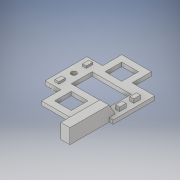
# Autodesk Inventor part: y-axis motor mount modified
Saved by Autodesk Inventor 2018 (Build 220112000, 112)
## iProperties
Created: 2018-02-05
Part Number: y-axis motor mount modified
Material: Generic
Document SubType Name: Modeling
Designer: junai
Density: 1 g/cm^3
Appearance: Default
Author: junai
Autodesk Inventor part; units mm, degrees
ref_plane "YZ Plane" through (0, 0, 0) normal (1, 0, 0) x (0, 1, 0)
ref_plane "XZ Plane" through (0, 0, 0) normal (0, 1, 0) x (-1, 0, 0)
ref_plane "XY Plane" through (0, 0, 0) normal (0, 0, 1) x (1, 0, 0)
sketch "Sketch1" plane through (0, 0, 0) normal (0, 1, 0) x (-1, 0, 0)
  circle A0 centre (0, 0) radius 2
  dimension "d0" = 4
  constraints: 1 centre point, 1 coincident
  measures "d0" diameter of A0
sketch "Sketch2" plane through (0, 0, 0) normal (0, 1, 0) x (-1, 0, 0)
  line L0 (-6, 8) -> (-21, 8)
  line L1 (-21, 8) -> (-21, -8)
  line L2 (-21, -8) -> (-6, -8)
  line L3 (-6, -8) -> (-6, 8)
  line L4 (0, 0) -> (-6, 0) construction
  line L5 (1.5, 13) -> (-1.5, 13)
  line L6 (-1.5, 13) -> (-1.5, 8)
  line L7 (-1.5, 8) -> (1.5, 8)
  line L8 (1.5, 8) -> (1.5, 13)
  line L9 (0, 0) -> (0, 8) construction
  line L10 (1.5, -13) -> (-1.5, -13)
  line L11 (-1.5, -13) -> (-1.5, -8)
  line L12 (-1.5, -8) -> (1.5, -8)
  line L13 (1.5, -8) -> (1.5, -13)
  line L14 (-13.5, 8) -> (-13.5, 16) construction
  line L15 (-13.5, -8) -> (-13.5, -16) construction
  line L16 (-6, 0) -> (4, 0) construction
  line L17 (-6, 0) -> (4, 0) construction
  line L18 (-6, 0) -> (4, 0) construction
  line L19 (-21, 0) -> (-46, 0) construction
  line L20 (6, 16) -> (-46, 16)
  line L21 (-46, 16) -> (-46, -16)
  line L22 (-46, -16) -> (6, -16)
  line L23 (6, -16) -> (6, 16)
  line L24 (-6, 0) -> (6, 0) construction
  line L25 (-6, 30.75) -> (-28.75, 30.75)
  line L26 (-28.75, 30.75) -> (-28.75, 8)
  line L27 (-28.75, 8) -> (-6, 8)
  line L28 (-6, 8) -> (-6, 30.75)
  line L29 (-11.3986, 8) -> (-11.3986, 8) construction
  line L30 (-6, -30.75) -> (-28.75, -30.75)
  line L31 (-28.75, -30.75) -> (-28.75, -8)
  line L32 (-28.75, -8) -> (-6, -8)
  line L33 (-6, -8) -> (-6, -30.75)
  line L34 (-11.3986, -8) -> (-11.3986, -8) construction
  line L35 (-39.6834, 6.855) -> (-42.6834, 6.855)
  line L36 (-42.6834, 6.855) -> (-42.6834, 1.855)
  line L37 (-42.6834, 1.855) -> (-39.6834, 1.855)
  line L38 (-39.6834, 1.855) -> (-39.6834, 6.855)
  dimension "d1" = 15
  dimension "d2" = 16
  dimension "d3" = 6
  dimension "d4" = 3
  dimension "d5" = 5
  dimension "d6" = 8
  dimension "d7" = 8
  dimension "d11" = 25
  dimension "d12" = 12
  dimension "d13" = 22.75
  dimension "d14" = 22.75
  dimension "d15" = 0
  dimension "d16" = 3
  dimension "d17" = 5
  constraints: 79 end point, 10 parallel, 10 symmetric about line, 8 horizontal, 7 midpoint, 6 perpendicular, 5 point on line, 2 vertical, 1 coincident, 1 collinear
  measures "d1" distance of L1.end L2.end
  measures "d2" distance of L0.end L1.end
  measures "d3" distance of L4.end L4.start
  measures "d4" distance of L7.end L6.end
  measures "d5" distance of L5.end L6.end
  measures "d6" distance of L4.start L9.end
  measures "d7" distance of L14.start L14.end
  measures "d11" distance of L19.end L19.start
  measures "d12" distance of L24.end L4.end
  measures "d13" distance of L27.end L26.end
  measures "d14" distance of L27.end L25.start
  measures "d15" distance of L29.start L29.end
  measures "d16" distance of L37.end L36.end
  measures "d17" distance of L35.end L36.end
sketch "Sketch3" plane through (0, 0, 0) normal (0, 1, 0) x (-1, 0, 0)
  point P0 (0, 0)
sketch "Sketch4" plane through (0, 0, 0) normal (0, 1, 0) x (-1, 0, 0)
  point P0 (0, 0)
sketch "Sketch5" plane through (0, 0, 0) normal (0, 1, 0) x (-1, 0, 0)
  point P0 (0, 0)
sketch "Sketch6" plane through (0, 0, 0) normal (0, 1, 0) x (-1, 0, 0)
  point P0 (0, 0)
extrude "Extrusion1" add sketch "Sketch2" along normal blind 3 contours L28 L20 L23 L22 L33 L3 | L0 L27 L26 L20 L28 | L1 L32 L31 L22 L21 L20 L26 L27 | L33 L22 L31 L32 L2 | L20 L26 L25 L28 | L33 L30 L31 L22 | L38 L37 L36 L35
sketch "Sketch7" plane through (0, 3, 0) normal (0, 1, 0) x (1, 0, 0)
  point P0 (0, 0)
extrude "Extrusion2" cut sketch "Sketch1" along normal blind 3
sketch "Sketch8" plane through (0, 3, 0) normal (0, 1, 0) x (1, 0, 0)
  line L0 (21, -8) -> (6, -8) projected
  line L1 (21, -8) -> (36, -8)
  line L2 (36, -8) -> (36, 8)
  line L3 (36, 8) -> (21, 8)
  line L4 (21, 8) -> (21, -8)
  line L5 (36, 0) -> (46, 0) construction
  line L6 (46, -16) -> (46, 16) construction
  line L7 (6, 8) -> (21, 8) construction
  point P0 (0, 0)
  dimension "d25" = 10
  constraints: 10 end point, 2 horizontal, 2 midpoint, 2 parallel, 1 collinear, 1 perpendicular
  measures "d25" distance of L5.start L5.end
extrude "Extrusion3" cut sketch "Sketch8" against normal blind 3
sketch "Sketch9" plane through (0, 3, 0) normal (0, 1, 0) x (1, 0, 0)
  line L0 (11, -25.75) -> (23.75, -25.75)
  line L1 (23.75, -25.75) -> (23.75, -13)
  line L2 (23.75, -13) -> (11, -13)
  line L3 (11, -13) -> (11, -25.75)
  line L4 (6, -30.75) -> (28.75, -30.75) construction
  line L5 (17.375, -30.75) -> (17.375, -25.75) construction
  line L6 (6, 0) -> (36, 0) construction
  line L7 (36, -8) -> (36, 8) construction
  line L8 (11, 25.75) -> (23.75, 25.75)
  line L9 (23.75, 25.75) -> (23.75, 13)
  line L10 (23.75, 13) -> (11, 13)
  line L11 (11, 13) -> (11, 25.75)
  line L12 (17.375, 30.75) -> (17.375, 25.75) construction
  line L13 (-1.5, -13) -> (-1.5, -8) projected
  line L14 (1.5, -8) -> (-1.5, -8) projected
  line L15 (-1.5, -13) -> (1.5, -13)
  line L16 (1.5, -13) -> (1.5, -8)
  line L17 (1.5, -8) -> (-1.5, -8)
  line L18 (-1.5, -8) -> (-1.5, -13)
  line L19 (-1.5, 8) -> (1.5, 8) projected
  line L20 (1.5, 8) -> (1.5, 13) projected
  line L21 (-1.5, 8) -> (1.5, 8)
  line L22 (1.5, 8) -> (1.5, 13)
  line L23 (1.5, 13) -> (-1.5, 13)
  line L24 (-1.5, 13) -> (-1.5, 8)
  point P0 (0, 0)
  dimension "d28" = 12.75
  dimension "d29" = 12.75
  dimension "d30" = 5
  constraints: 38 end point, 6 parallel, 6 symmetric about line, 4 perpendicular, 3 horizontal, 3 midpoint
  measures "d28" distance of L2.end L1.end
  measures "d29" distance of L0.end L1.end
  measures "d30" distance of L5.end L5.start
extrude "Extrusion4" add sketch "Sketch9" along normal mid plane 3 contours L13 L14 L16 L15 | L24 L23 L20 L19
sketch "Sketch10" plane through (0, 3, 0) normal (0, 1, 0) x (1, 0, 0)
  line L0 (40, -8) -> (43, -8)
  line L1 (43, -8) -> (43, -3)
  line L2 (43, -3) -> (40, -3)
  line L3 (40, -3) -> (40, -8)
  line L4 (36, -8) -> (6, -8) projected
  line L5 (36, 8) -> (36, -8) construction
  line L6 (36, -5.7652) -> (40, -5.7652) construction
  line L7 (36, 0) -> (46, 0) construction
  line L8 (46, -16) -> (46, 16) construction
  line L9 (40, 8) -> (43, 8)
  line L10 (43, 8) -> (43, 3)
  line L11 (43, 3) -> (40, 3)
  line L12 (40, 3) -> (40, 8)
  point P0 (0, 0)
  dimension "d33" = 3
  dimension "d34" = 5
  dimension "d35" = 4
  constraints: 20 end point, 4 symmetric about line, 2 midpoint, 2 parallel, 2 perpendicular, 2 point on line, 1 collinear, 1 horizontal
  measures "d33" distance of L2.end L1.end
  measures "d34" distance of L0.end L1.end
  measures "d35" distance of L6.start L6.end
extrude "Extrusion5" add sketch "Sketch10" along normal blind 3
sketch "Sketch11" plane through (0, 3, 0) normal (0, 1, 0) x (1, 0, 0)
  line L0 (36, 8) -> (36, -8) construction
  line L1 (36, -8) -> (36, -16) construction
  line L2 (28.75, -16) -> (46, -16) construction
  line L3 (36, -16) -> (43, -16)
  line L4 (43, -16) -> (43, -46)
  line L5 (43, -46) -> (36, -46)
  line L6 (36, -46) -> (36, -16)
  point P0 (0, 0)
  dimension "d38" = 7
  dimension "d39" = 30
  constraints: 10 end point, 2 parallel, 1 horizontal, 1 perpendicular, 1 point on line, 1 vertical
  measures "d38" distance of L4.end L5.end
  measures "d39" distance of L3.end L4.end
extrude "Extrusion6" add sketch "Sketch11" along normal blind 8.35 and the other way blind 3
sketch "Sketch12" plane through (43, 0, 46) normal (1, 0, 0) x (0, 0, -1)
  point P0 (46, 0)
sketch "Sketch13" plane through (43, 3, 16) normal (0, 0, -1) x (-1, 0, 0)
  point P0 (43, -3)
draft "FaceDraft1" angle 30 pull direction (0, 1, 0) faces at (38.3333, 8.5667, 16) fixed edges at (39.5, 11.35, 16)
sketch "Sketch14" plane through (0, 3, 0) normal (0, 1, 0) x (1, 0, 0)
  line L0 (11, -25.75) -> (23.75, -25.75)
  line L1 (23.75, -25.75) -> (23.75, -13)
  line L2 (23.75, -13) -> (11, -13)
  line L3 (11, -13) -> (11, -25.75)
  line L4 (6, -30.75) -> (28.75, -30.75) construction
  line L5 (17.375, -25.75) -> (17.375, -30.75) construction
  line L6 (28.75, -30.75) -> (28.75, -16) construction
  line L7 (6, -16) -> (6, -30.75) construction
  line L8 (36, -8) -> (6, -8) construction
  line L9 (36, -8) -> (6, -8) construction
  line L10 (6, -30.75) -> (28.75, -30.75) construction
  line L11 (28.75, -30.75) -> (28.75, -8) construction
  line L12 (28.75, -8) -> (6, -8) construction
  line L13 (6, -8) -> (6, -30.75) construction
  line L14 (28.75, -19.375) -> (23.75, -19.375) construction
  line L15 (6, 8) -> (6, -8) construction
  line L16 (6, 0) -> (36, 0) construction
  line L17 (36, -8) -> (36, 8) construction
  line L18 (11, 25.75) -> (23.75, 25.75)
  line L19 (23.75, 25.75) -> (23.75, 13)
  line L20 (23.75, 13) -> (11, 13)
  line L21 (11, 13) -> (11, 25.75)
  point P0 (0, 0)
  dimension "d46" = 12.75
  dimension "d47" = 12.75
  constraints: 30 end point, 8 midpoint, 5 parallel, 4 symmetric about line, 3 horizontal, 3 perpendicular, 1 point on line, 1 vertical
  measures "d46" distance of L2.end L1.end
  measures "d47" distance of L0.end L1.end
extrude "Extrusion7" cut sketch "Sketch14" against normal blind 8.35
body "Solid1"
